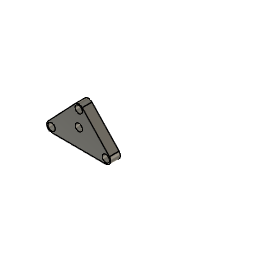
digiObscura Camera_TripodMount (Autodesk Fusion 360 design; units mm, degrees)
Autodesk Fusion 360 part; units mm, degrees
sketch "Sketch1" plane through (0, -52, 0) normal (0, -1, 0) x (1, 0, 0)
  circle A0 centre (-22.4654, 29.7532) radius 2.1
  circle A1 centre (0, 53.5) radius 2.1
  circle A2 centre (22.4552, 29.5809) radius 2.1
  line L0 (50, -12.6) -> (50, 56.6)
  line L1 (50, 56.6) -> (-50, 56.6)
  line L2 (-50, 56.6) -> (-50, -12.6)
  line L3 (-50, -12.6) -> (50, -12.6)
  circle A3 centre (0, 53.5) radius 4
  circle A4 centre (-22.4654, 29.7532) radius 4
  circle A5 centre (22.4552, 29.5809) radius 4
  line L4 (-25.3712, 32.5022) -> (-2.9057, 56.2489)
  line L5 (2.9163, 56.2378) -> (25.3715, 32.3187)
  line L6 (22.4399, 25.5809) -> (-22.4808, 25.7532)
  circle A6 centre (-22.4654, 29.7532) radius 1.65
  circle A7 centre (0, 53.5) radius 1.65
  circle A8 centre (22.4552, 29.5809) radius 1.65
  circle A9 centre (0.0409, 40.6669) radius 2.95
  dimension "d98" = 8
  dimension "d99" = 8
  dimension "d100" = 8
  dimension "d101" = 3.3
  dimension "d102" = 3.3
  dimension "d103" = 3.3
  dimension "d104" = 5.9
  dimension "d157" = 15
  constraint concentric A1 A3
  constraint concentric A0 A4
  constraint concentric A2 A5
  constraint coincident A4 L4.start
  constraint coincident A3 L4.end
  constraint tangent A3 L4
  constraint coincident A3 L5.start
  constraint coincident A5 L5.end
  constraint tangent A5 L5
  constraint coincident A5 L6.start
  constraint coincident A4 L6.end
  constraint tangent A4 L6
  constraint tangent A4 L4
  constraint tangent A3 L5
  constraint tangent A5 L6
  constraint concentric A4 A6
  constraint concentric A3 A7
  constraint concentric A5 A8
  measures "d98" diameter of A4
  measures "d99" diameter of A3
  measures "d100" diameter of A5
  measures "d101" diameter of A6
  measures "d102" diameter of A7
  measures "d103" diameter of A8
  measures "d104" diameter of A9
  measures "d157" distance of L6 A9.centre
extrude "Extrude1" add sketch "Sketch1" along normal blind 8 contours A0 | A1 | A2 | L1 A3 | L1 A3 | A3 A4 A5 L4 L5 L6 | A5 | A4
sketch "Sketch2" plane through (0, -60, 0) normal (0, -1, 0) x (1, 0, 0)
  circle A0 centre (0.0409, 40.6669) radius 2.95
  circle A1 centre (-22.4654, 29.7532) radius 1.65
  circle A2 centre (0, 53.5) radius 1.65
  circle A3 centre (22.4552, 29.5809) radius 1.65
  arc A4 (2.9163, 56.2378) -> (-2.9057, 56.2489) centre (0, 53.5) ccw
  line L0 (-2.9057, 56.2489) -> (-25.3712, 32.5022)
  arc A5 (-25.3712, 32.5022) -> (-22.4808, 25.7532) centre (-22.4654, 29.7532) ccw
  line L1 (-22.4808, 25.7532) -> (22.4399, 25.5809)
  arc A6 (22.4399, 25.5809) -> (25.3715, 32.3187) centre (22.4552, 29.5809) ccw
  line L2 (25.3715, 32.3187) -> (2.9163, 56.2378)
  circle A7 centre (22.4552, 29.5809) radius 3
  circle A8 centre (-22.4654, 29.7532) radius 3
  circle A9 centre (0, 53.5) radius 3
  dimension "d107" = 6
  dimension "d108" = 6
  dimension "d109" = 6
  constraint concentric A3 A7
  constraint concentric A1 A8
  constraint concentric A2 A9
  measures "d107" diameter of A7
  measures "d108" diameter of A9
  measures "d109" diameter of A8
extrude "Extrude2" cut sketch "Sketch2" against normal blind 5 contours A7 | A8 | A9
